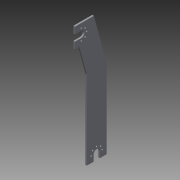
# Autodesk Inventor part: Flame
Saved by Autodesk Inventor 2013 (Build 170138000, 138)
## iProperties
Created: 2014-04-16
Part Number: Flame
Material: 一般
Document SubType Name: Modeling
Designer: andou
Density: 1 g/cm^3
Author: andou
Autodesk Inventor part; units mm, degrees
ref_plane "YZ Plane" through (0, 0, 0) normal (1, 0, 0) x (0, 1, 0)
ref_plane "XZ Plane" through (0, 0, 0) normal (0, 1, 0) x (-1, 0, 0)
ref_plane "XY Plane" through (0, 0, 0) normal (0, 0, 1) x (1, 0, 0)
sketch "スケッチ1" plane through (0, 0, 0) normal (1, 0, 0) x (0, 1, 0)
  line L0 (-20, 80) -> (20, 80)
  line L1 (20, 80) -> (20, -80)
  line L2 (20, -80) -> (-20, -80)
  line L3 (-20, -80) -> (-20, 80)
  point P0 (0, 0)
  dimension "d0" = 40
  dimension "d2" = 160
  dimension "d3" = 80
  dimension "d4" = 20
  constraints: 8 end point, 2 parallel, 1 horizontal, 1 perpendicular
  measures "d0" distance of L0.start L0.end
  measures "d2" distance of L2.end L0.start
  measures "d3" distance from line of point (0, 0) L0
  measures "d4" distance from line of L1 point (0, 0)
extrude "押し出し1" add sketch "スケッチ1" along normal blind 2
sketch "スケッチ2" plane through (2, 0, 0) normal (1, 0, 0) x (0, 0, -1)
  line L0 (-80, 20) -> (-80, -20) projected
  line L1 (-80, -20) -> (80, -20) projected
  line L2 (80, -20) -> (80, 20) projected
  line L3 (80, 20) -> (-80, 20) projected
  line L4 (-80, 3.923) -> (-20, 20)
  line L5 (-55, -20) -> (-55, -14.3782)
  line L6 (-55, -14.3782) -> (-20, -5)
  line L7 (-20, -5) -> (80, -5)
  point P0 (0, 0)
  dimension "d7" = 25
  dimension "d8" = 165
  dimension "d9" = 15
  dimension "d10" = 100
  dimension "d11" = 100
  dimension "d12" = 25
  constraints: 8 end point, 4 point on line, 2 perpendicular
  measures "d7" distance between parallel lines of L3 L7
  measures "d8" angle of L7 L6
  measures "d9" angle of L3 L4
  measures "d10" distance from line of L2 L4.end
  measures "d11" distance of L6.end L7.end
  measures "d12" distance between parallel lines of L0 L5
extrude "押し出し2" cut sketch "スケッチ2" against normal blind 2 contours L4 L3 L2 L7 L6 L5 L1 L0 keep common part
sketch "スケッチ3" plane through (2, 0, 0) normal (1, 0, 0) x (0, 0, -1)
  line L0 (80, -5) -> (-20, -5) projected
  line L1 (80, -5) -> (80, 20) projected
  line L2 (80, 20) -> (-20, 20) projected
  line L3 (-80, 3.923) -> (-20, 20) projected
  line L4 (-80, 3.923) -> (-80, -20) projected
  line L5 (-80, -20) -> (-55, -20) projected
  line L6 (-55, -14.3782) -> (-55, -20) projected
  line L7 (-20, -5) -> (-55, -14.3782) projected
  line L8 (-71.5, -20) -> (-63.5, -20)
  line L9 (-63.5, -20) -> (-63.5, -12)
  line L10 (-71.5, -12) -> (-71.5, -20)
  line L11 (80, 11.5) -> (72, 11.5)
  line L12 (72, 3.5) -> (80, 3.5)
  line L13 (80, 3.5) -> (80, 11.5)
  arc A0 (-63.5, -12) -> (-71.5, -12) centre (-67.5, -12) ccw
  arc A1 (72, 11.5) -> (72, 3.5) centre (72, 7.5) ccw
  point P0 (0, 0)
  dimension "d18" = 8
  dimension "d19" = 12.5
  dimension "d20" = 8
  dimension "d21" = 12.5
  dimension "d23" = 8
  dimension "d24" = 4
  dimension "d25" = 8
  dimension "d26" = 8
  dimension "d27" = 8
  constraints: 12 end point, 4 point on circle, 2 centre point, 2 horizontal, 2 parallel, 2 point on line, 1 equal radius, 1 perpendicular
  measures "d18" distance between parallel lines of L9 L10
  measures "d19" distance from line of L6 A0.centre
  measures "d20" distance between parallel lines of L11 L12
  measures "d21" distance from line of L0 A1.centre
  measures "d23" distance from line of L8 A0.centre
  measures "d24" radius of A0
  measures "d25" distance of L8.end L9.end
  measures "d26" distance from line of L1 A1.centre
  measures "d27" distance of L11.start L11.end
extrude "押し出し3" cut sketch "スケッチ3" against normal blind 2 contours L0 L7 L6 L5 L9 A0 L10 L4 L3 L2 L1 L11 A1 L12 keep common part
sketch "スケッチ4" plane through (2, 0, 0) normal (1, 0, 0) x (0, 0, -1)
  arc A0 (72, 11.5) -> (72, 3.5) centre (72, 7.5) ccw projected
  line L0 (80, 11.5) -> (80, 20) projected
  line L1 (-80, -20) -> (-71.5, -20) projected
  arc A1 (-63.5, -12) -> (-71.5, -12) centre (-67.5, -12) ccw projected
  circle A2 centre (-74.5, -12) radius 1
  circle A3 centre (72, 14.5) radius 1
  point P0 (0, 0)
  dimension "d30" = 8
  dimension "d31" = 7
  dimension "d32" = 2
  dimension "d33" = 8
  dimension "d34" = 7
  constraints: 2 centre point, 1 equal radius
  measures "d30" distance from line of A2.centre L1
  measures "d31" distance of A1.centre A2.centre
  measures "d32" diameter of A2
  measures "d33" distance from line of L0 A3.centre
  measures "d34" distance of A3.centre A0.centre
hole "穴1" at (2, -12, 74.5) at (2, 14.5, -72) direction (-1, 0, 0) diameter 2 end through all
pattern_circular "円形状パターン1" count 5 over 180 about axis through (2, -12, 67.5) along (-1, 0, 0) of "穴1"
pattern_circular "円形状パターン2" count 5 over 180 about axis through (2, 7.5, -72) along (1, 0, 0) of "穴1"
